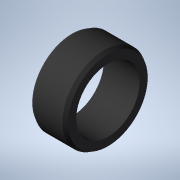
# Autodesk Inventor part: 8210495 ZBH-7
Saved by Autodesk Inventor 2021 (Build 250183000, 183)
## iProperties
Created: 2026-04-25
Part Number: 8210495 ZBH-7
Material: Generic
Catalog Web Link: www.3dfindit.com
Description: ZBH2-centring sleeve
Vendor: FESTO
Document SubType Name: Modeling
Designer: psAdmin
Manufacturer: FESTO
Mass: 0.4 g
Surface Area: 1.43005 cm^2
Volume: 0.0481442 cm^3
Density: 1 g/cm^3
Appearance: PSOLRGB-176-176-176
Category: PARTsolutions
Company: FESTO
Title: 8210495 ZBH-7
Author: Cadenas PARTsolutions
Comments: centring sleeve
PSOL_IDENT_0: {$CADENAS_DATA/23d-libs/festo/parts/z/zbh/zbh2.prj},164 {VTYP=3D},{NB=8210495 ZBH-7},{LINA=8210495 Z
PSOL_IDENT_1: BH-7},{NN=ZBH2},{DATE=24.03.2026 10:11:30},{GEOMDATE=24.03.2026 10:11:00},{VERSION=},{LINEID=20},{WB
PSOL_IDENT_2: VAR=},{WBNUMERIC=}  {NB=8210495 ZBH-7},{LINA=8210495 ZBH-7},{KT=DUMMY},{TNR=8210495},{TYP=ZBH-7},{B1=
PSOL_IDENT_3: 3.000},{D1=7.000},{D2=5.300},{F=0.300},{CNSMASSEXACT=0.0004},{GTIN=4052568652715}
NB: 8210495 ZBH-7
NN: ZBH2
NT: centring sleeve
NBSYN: $TNR. $TYP.
LINA: 8210495 ZBH-7
CATALOG: Festo
TNR: 8210495
TYP: ZBH-7
B1: 3
D1: 7
D2: 5.3
F: 0.3
CNSMASSEXACT: 0.0004
GTIN: 4052568652715
SUPPLIER: FESTO
ARTICLENO: 8210495 ZBH-7
BOMINFO: 8210495 ZBH-7
CREATOR: CADENAS GmbH
Autodesk Inventor part; units mm, degrees
sketch "Sketch_1" plane through (0, 0, 0) normal (0, 0, 1) x (1, 0, 0)
  line L0 (3, 0) -> (0, 0)
  line L1 (0, 2.65) -> (3, 2.65)
  line L2 (3, 2.65) -> (3, 3.3268)
  line L3 (3, 3.3268) -> (2.7, 3.5)
  line L4 (2.7, 3.5) -> (0.3, 3.5)
  line L5 (0.3, 3.5) -> (0, 3.3268)
  line L6 (0, 3.3268) -> (0, 2.65)
  constraints: 14 end point
revolve "Revolution1" add sketch "Sketch_1" angle 360 about axis through (3, 0, 0) along (-1, 0, 0)
ref_plane "ANBAU_XY" through (0, 0, 0) normal (1, 0, 0) x (0, 0, -1)
ref_plane "ANBAU_YZ" through (0, 0, 0) normal (0, 0, -1) x (0, 1, 0)
ref_plane "ANBAU_ZX" through (0, 0, 0) normal (0, 1, 0) x (1, 0, 0)
ref_plane "INSERT_XY" through (0, 0, 0) normal (1, 0, 0) x (0, 0, -1)
ref_plane "INSERT_YZ" through (0, 0, 0) normal (0, 0, -1) x (0, 1, 0)
ref_plane "INSERT_ZX" through (0, 0, 0) normal (0, 1, 0) x (1, 0, 0)
ref_plane "SCHRAUBE_PUNKT_XY" through (3, 0, 0) normal (1, 0, 0) x (0, 0, -1)
ref_plane "SCHRAUBE_PUNKT_YZ" through (3, 0, 0) normal (0, 0, -1) x (0, 1, 0)
ref_plane "SCHRAUBE_PUNKT_ZX" through (3, 0, 0) normal (0, 1, 0) x (1, 0, 0)
body "Solid1"
